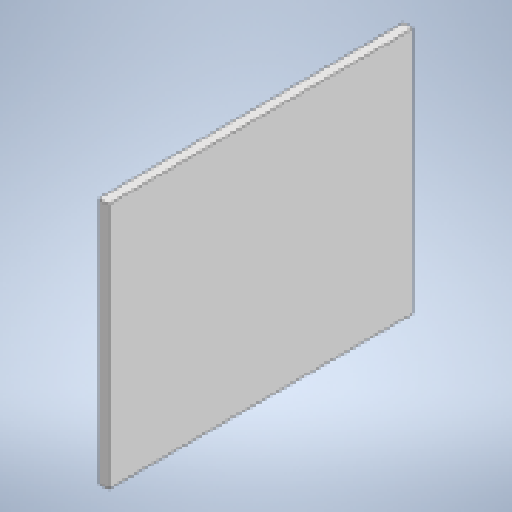
# Autodesk Inventor part: door
Saved by Autodesk Inventor 2023 (Build 270158030, 158C)
## iProperties
Created: 2024-04-01
Part Number: door
Material: Generic
Document SubType Name: Modeling
Designer: Imogen Heard
Density: 1 g/cm^3
Appearance: Default
Author: Imogen Heard
Autodesk Inventor part; units mm, degrees
ref_plane "YZ Plane" through (0, 0, 0) normal (1, 0, 0) x (0, 1, 0)
ref_plane "XZ Plane" through (0, 0, 0) normal (0, 1, 0) x (-1, 0, 0)
ref_plane "XY Plane" through (0, 0, 0) normal (0, 0, 1) x (1, 0, 0)
sketch "Sketch1" plane through (0, 0, 0) normal (0, 0, 1) x (1, 0, 0)
  circle A0 centre (-0.4774, -6.0596) radius 2.15 projected
  circle A1 centre (-0.4774, -6.0596) radius 2.8
  line L0 (-3.2774, -6.0596) -> (2.3226, -6.0596)
  line L1 (2.3226, -6.0596) -> (2.3226, -1.0596)
  line L2 (2.3226, -1.0596) -> (-3.2774, -1.0596)
  line L3 (-3.2774, -1.0596) -> (-3.2774, -6.0596)
  point P0 (0, 0)
  dimension "d1" = 5.6
  dimension "d2" = 5
  constraints: 8 end point, 2 parallel, 1 horizontal, 1 perpendicular, 3 other
  measures "d2" distance between parallel lines of L0 L2
extrude "Extrusion1" add sketch "Sketch1" along normal blind 10 contours L0 A1 A0 | A0 L0 A1 | A1 L3 L2 L1
sketch "Sketch2" plane through (-3.2774, -1.0596, 0) normal (0, 1, 0) x (1, 0, 0)
  line L0 (0, 49.3) -> (14, 49.3)
  line L1 (14, 49.3) -> (14, -439.7)
  line L2 (14, -439.7) -> (0, -439.7)
  line L3 (0, -439.7) -> (0, 49.3)
  line L4 (-5.1549, -390) -> (-5.1549, -380) projected
  line L5 (-5.1549, -380) -> (9.8, -380) projected
  line L6 (9.8, -380) -> (9.8, -390) projected
  line L7 (9.8, -390) -> (-5.1549, -390) projected
  line L8 (-5.1549, 0) -> (-5.1549, 10) projected
  line L9 (-5.1549, 10) -> (9.8, 10) projected
  line L10 (9.8, 10) -> (9.8, 0) projected
  line L11 (9.8, 0) -> (-5.1549, 0) projected
  line L12 (10.8, -425.4) -> (10.8, 35) projected
  line L13 (10.8, 35) -> (371.2, 35) projected
  line L14 (371.2, 35) -> (371.2, -425.4) projected
  line L15 (371.2, -425.4) -> (10.8, -425.4) projected
  line L16 (388.5, -442.7) -> (388.5, 52.3) projected
  line L17 (388.5, 52.3) -> (-6.5, 52.3) projected
  line L18 (-6.5, 52.3) -> (-6.5, -442.7) projected
  line L19 (-6.5, -442.7) -> (388.5, -442.7) projected
  point P0 (3.2774, 0)
  point P1 (0, -10)
  dimension "d5" = 14
  dimension "d6" = 489
  dimension "d7" = 3
  dimension "d8" = 3
  constraints: 8 end point, 2 parallel, 1 horizontal, 1 perpendicular, 1 vertical alignment
  measures "d5" distance between parallel lines of L1 L3
  measures "d6" distance between parallel lines of L0 L2
  measures "d7" distance between parallel lines of L19 L2
  measures "d8" distance between parallel lines of L17 L0
extrude "Extrusion2" add sketch "Sketch2" along normal blind 1.6 contours L0 L1 L13 L12 L15 L2 L3 L7 L6 L5 L11 L10 L9 | L9 L10 L11 L3 | L1 L15 L12 L13 | L5 L6 L7 L3
sketch "Sketch3" plane through (10.7226, -1.0596, 439.7) normal (1, 0, 0) x (0, 0, -1)
  line L0 (489, 0) -> (489, 1.6) projected
  line L1 (489, 1.6) -> (0, 1.6)
  line L2 (0, 1.6) -> (0, -394.4)
  line L3 (0, -394.4) -> (489, -394.4)
  line L4 (489, -394.4) -> (489, 1.6)
  point P0 (439.7, 1.0596)
  dimension "d11" = 396
  constraints: 8 end point, 2 parallel, 1 horizontal, 1 perpendicular
  measures "d11" distance between parallel lines of L3 L1
extrude "Extrusion3" add sketch "Sketch3" along normal blind 1.6
sketch "Sketch4" plane through (10.7226, -1.0596, 439.7) normal (-1, 0, 0) x (0, 0, 1)
  line L0 (0, 0) -> (-1.6, 0)
  line L1 (-1.6, 0) -> (-1.6, -394.4)
  line L2 (-1.6, -394.4) -> (0, -394.4)
  line L3 (0, -394.4) -> (0, 0)
  line L4 (-1.6, -392.8) -> (-489, -392.8)
  line L5 (-489, -392.8) -> (-489, -394.4)
  line L6 (-489, -394.4) -> (-1.6, -394.4)
  line L7 (-1.6, -394.4) -> (-1.6, -392.8)
  line L8 (-487.4, 0) -> (-489, 0)
  line L9 (-489, 0) -> (-489, -394.4)
  line L10 (-489, -394.4) -> (-487.4, -394.4)
  line L11 (-487.4, -394.4) -> (-487.4, 0)
  point P0 (-439.7, 1.0596)
  point P1 (0, 0)
  point P2 (-487.4, -392.8)
  point P3 (-489, -392.8)
  point P4 (-1.6, -394.4)
  dimension "d14" = 1.6
  dimension "d15" = 1.6
  dimension "d16" = 1.6
  constraints: 24 end point, 6 coincident, 6 parallel, 3 horizontal, 3 perpendicular, 2 point on line, 1 horizontal alignment
  measures "d14" distance between parallel lines of L9 L11
  measures "d15" distance between parallel lines of L6 L4
  measures "d16" distance between parallel lines of L3 L1
extrude "Extrusion4" add sketch "Sketch4" along normal up to surface (14 mm away)
body "Solid1"
